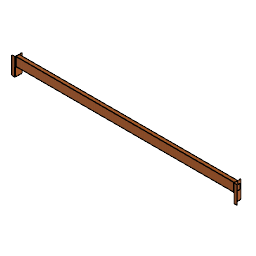
_Cross Bar.9fb02594-36a0-4474-9139-e6fe5210b81d (Autodesk Fusion 360 design; units mm, degrees)
Autodesk Fusion 360 part; units mm, degrees
(part 1 of 2)
sketch "Sketch1" plane through (0, 0, 0) normal (0, 1, 0) x (1, 0, 0)
  line L0 (-1250.95, 0) -> (0, 0)
  line L1 (-1257.3, 6.35) -> (-1257.3, 203.2)
  line L2 (-1257.3, 203.2) -> (-1216.025, 203.2)
  line L3 (-1257.3, 6.35) -> (-1250.95, 0)
  line L4 (-1216.025, 0) -> (-1216.025, 101.6)
  line L5 (-1216.025, 101.6) -> (-1216.025, 203.2)
  line L6 (0, 0) -> (0, -58.9173) construction
  line L7 (-1216.025, 101.6) -> (0, 101.6)
  line L8 (0, 0) -> (0, -58.9173) construction
  line L9 (1216.025, 0) -> (1216.025, 101.6)
  line L10 (1216.025, 101.6) -> (1216.025, 203.2)
  line L11 (1250.95, 0) -> (0, 0)
  line L12 (1257.3, 6.35) -> (1257.3, 203.2)
  line L13 (1257.3, 6.35) -> (1250.95, 0)
  line L14 (1257.3, 203.2) -> (1216.025, 203.2)
  line L15 (1216.025, 101.6) -> (0, 101.6)
  dimension "d3" = 41.275
  dimension "d6" = 101.6
  constraint coincident L0.end L6.start
  constraint horizontal L0
  constraint perpendicular L0 L1
  constraint perpendicular L1 L2
  constraint coincident L0 L6.start
  constraint coincident L0 L4.start
  constraint perpendicular L0 L4
  constraint perpendicular L2 L5
  constraint perpendicular L0 L6
  constraint coincident L6 L0.end
  constraint perpendicular L4 L7
  constraint symmetric L0.end L6 L8.start
  constraint symmetric L1.end L6 L12.end
  constraint symmetric L2.end L6 L10.end
  constraint symmetric L1.start L6 L12.start
  constraint symmetric L0.start L6 L11.start
  constraint symmetric L4.start L6 L9.start
  constraint symmetric L4.end L6 L9.end
  constraint symmetric L8.end L6 L6.end
  constraint symmetric L6 L0.end L8.start
  constraint symmetric L6 L7.end L15.end
  measures "d3" distance of L1.end L2.end
  measures "d6" distance of L4.start L4.end
extrude "Extrude1" add sketch "Sketch1" against normal blind 3.175 contours L0 L1 L2 L3 L4 L5 | L9 L10 L11 L12 L13 L14 makes body 1 at (-1229.7833, 0, -69.85) makes body 2 at (1229.7833, 0, -69.85)
ref_plane "WorkPlane1" through (1236.6625, 3.175, -101.6) normal (0, -1, 0) x (0, 0, -1)
sketch "Sketch2" plane through (0, 3.175, 0) normal (0, -1, 0) x (-1, 0, 0)
  line L0 (-1257.3, 6.35) -> (-1257.3, 203.2)
  line L1 (-1216.025, 0) -> (-1216.025, 101.6)
  line L2 (-1216.025, 101.6) -> (0, 101.6)
  line L3 (-1250.95, 0) -> (0, 0)
  line L4 (-1257.3, 6.35) -> (-1250.95, 0)
  line L5 (-1216.025, 101.6) -> (-1216.025, 203.2)
  line L6 (-1257.3, 203.2) -> (-1216.025, 203.2)
  line L7 (1216.025, 101.6) -> (0, 101.6)
  line L8 (1250.95, 0) -> (0, 0)
  line L9 (1257.3, 6.35) -> (1250.95, 0)
  line L10 (1257.3, 6.35) -> (1257.3, 203.2)
  line L11 (1216.025, 0) -> (1216.025, 101.6)
  line L12 (1257.3, 203.2) -> (1216.025, 203.2)
  line L13 (1216.025, 101.6) -> (1216.025, 203.2)
extrude "Extrude2" add sketch "Sketch2" against normal blind 42.545 separate body contours L1 L2 L3 L7 L8 L11 makes body 3
sketch "Sketch3" plane through (0, 0, 0) normal (0, 0, 1) x (-1, 0, 0)
  line L0 (1216.025, -3.175) -> (-1216.025, -3.175)
  line L1 (-1216.025, -3.175) -> (-1216.025, -45.72)
  line L2 (-1216.025, -45.72) -> (1216.025, -45.72)
  line L3 (1216.025, -45.72) -> (1216.025, -3.175)
  line L4 (-1250.95, 0) -> (-1216.025, 0)
  line L5 (-1216.025, 0) -> (-1216.025, 3.175)
  line L6 (-1216.025, 3.175) -> (-1250.95, 3.175)
  line L7 (-1250.95, 3.175) -> (-1250.95, 0)
  line L8 (-1216.025, -3.175) -> (-1212.215, -3.175)
  line L9 (-1216.025, 3.175) -> (-1212.215, -3.175)
  line L10 (-1216.025, 0) -> (-1216.025, -3.175)
  line L11 (-1250.95, 0) -> (-1250.95, 3.175)
  line L12 (1219.2, -45.72) -> (-1219.2, -45.72)
  line L13 (-1219.2, -45.72) -> (-1219.2, 0)
  line L14 (0, -3.175) -> (0, -45.72)
  line L15 (0, -24.4475) -> (-1216.025, -24.4475)
  line L16 (-1257.3, 3.175) -> (-1250.95, 3.175)
  line L17 (-1257.3, 0) -> (-1257.3, 3.175)
  line L18 (-1257.3, 0) -> (-1250.95, 0)
  line L19 (-1250.95, 0) -> (-1250.95, 3.175)
  line L20 (-1250.95, 3.175) -> (-1257.3, 3.175)
  line L21 (-1257.3, 3.175) -> (-1257.3, 0)
  line L22 (-1216.025, -3.175) -> (1216.025, -3.175)
  line L23 (0, -24.4475) -> (1216.025, -24.4475)
  line L24 (1216.025, -3.175) -> (1216.025, -45.72)
  line L25 (1216.025, 0) -> (1216.025, 3.175)
  line L26 (-1219.2, -45.72) -> (1219.2, -45.72)
  line L27 (1257.3, 0) -> (1250.95, 0)
  line L28 (1216.025, -45.72) -> (-1216.025, -45.72)
  line L29 (1250.95, 3.175) -> (1250.95, 0)
  line L30 (1257.3, 3.175) -> (1250.95, 3.175)
  line L31 (1216.025, -3.175) -> (1212.215, -3.175)
  line L32 (1250.95, 3.175) -> (1257.3, 3.175)
  line L33 (1250.95, 0) -> (1216.025, 0)
  line L34 (1216.025, 3.175) -> (1250.95, 3.175)
  line L35 (1216.025, 3.175) -> (1212.215, -3.175)
  line L36 (1250.95, 0) -> (1250.95, 3.175)
  line L37 (1250.95, 0) -> (1250.95, 3.175)
  line L38 (1216.025, 0) -> (1216.025, -3.175)
  line L39 (1257.3, 0) -> (1257.3, 3.175)
  line L40 (1219.2, -45.72) -> (1219.2, 0)
  line L41 (1257.3, 3.175) -> (1257.3, 0)
  point P0 (0, -45.72)
  dimension "d12" = 3.81
  dimension "d13" = 2438.4
  constraint coincident L0.end L1.start
  constraint perpendicular L1 L8
  constraint coincident L5.end L6.start
  constraint coincident L4.end L5.start
  constraint coincident L4.start L7.end
  constraint coincident L6.end L7.start
  constraint midpoint L12 P0
  constraint coincident L2 P0
  constraint parallel L2 L12
  constraint coincident L4 L13.end
  constraint perpendicular L4 L13
  constraint midpoint L0 L14.start
  constraint coincident P0 L14.end
  constraint perpendicular L12 L14
  constraint midpoint L14 L15.start
  constraint midpoint L1 L15.end
  constraint symmetric L0.start L14 L0.end
  constraint symmetric L0.end L14 L0.start
  constraint symmetric L1.end L14 L2.end
  constraint symmetric L2.end L14 L1.end
  constraint symmetric L4.start L14 L27.end
  constraint symmetric L4.end L14 L25.start
  constraint symmetric L5.end L14 L25.end
  constraint symmetric L6.end L14 L29.start
  constraint symmetric L8.end L14 L31.end
  constraint symmetric L12.start L14 L12.end
  constraint symmetric L12.end L14 L12.start
  constraint symmetric L13.end L14 L40.end
  constraint symmetric L14 L15.start L23.start
  constraint symmetric L14 L15.end L23.end
  constraint symmetric L14 L16.start L30.start
  constraint symmetric L14 L6.end L29.start
  constraint symmetric L14 L17.start L27.start
  constraint symmetric L14 L4.start L27.end
  measures "d12" distance of L0.end L8.end
  measures "d13" distance of L12.start L12.end
extrude "Extrude3" add sketch "Sketch3" against normal blind 203.2 contours L3 L12 L24 L26 L33 L38 L40 | L0 L22 L25 L31 L35 L38 | L0 L5 L8 L9 L10 L22 | L1 L4 L10 L12 L13 L26 bodies 1 2 3
delete_face "DeleteFace1" 1 faces at (1213.485, 3.175, -169.3333) on bodies 1
delete_face "DeleteFace2" 1 faces at (-1214.755, 3.175, -135.4667) on bodies 1
sketch "Sketch4" plane through (0, 45.72, 0) normal (0, 1, 0) x (-1, 0, 0)
  line L0 (1219.2, 0) -> (-1219.2, 0)
  line L1 (-1219.2, 0) -> (-1219.2, -203.2)
  line L2 (-1219.2, -203.2) -> (-1216.025, -203.2)
  line L3 (-1216.025, -203.2) -> (-1216.025, -101.6)
  line L4 (-1216.025, -101.6) -> (1216.025, -101.6)
  line L5 (1216.025, -101.6) -> (1216.025, -203.2)
  line L6 (1216.025, -203.2) -> (1219.2, -203.2)
  line L7 (1219.2, -203.2) -> (1219.2, 0)
  line L8 (0, 0) -> (0, -41.91)
  line L9 (-1219.2, -41.91) -> (1219.2, -41.91)
  line L10 (1216.025, -101.6) -> (1219.2, -101.6)
  line L11 (1219.2, -101.6) -> (-1219.2, -101.6)
  dimension "d16" = 41.91
  constraint coincident L8.start origin
  constraint perpendicular L0 L8
  constraint midpoint L8.end L9
  constraint coincident L7 L9.end
  constraint perpendicular L7 L9
  constraint coincident L4.end L5.start
  constraint midpoint L7 L10.end
  constraint midpoint L1 L11.end
  measures "d16" distance of L8.start L8.end
extrude "Extrude4" add sketch "Sketch4" along normal blind 25.4 contours L1 L4 L7 L9 L10 L11 bodies 1
sketch "Sketch5" plane through (1219.2, 0, 0) normal (1, 0, 0) x (0, 1, 0)
  line L0 (45.72, 0) -> (0, 0)
  line L1 (0, 0) -> (0, -203.2)
  line L2 (0, -203.2) -> (45.72, -203.2)
  line L3 (45.72, -203.2) -> (45.72, -101.6)
  line L4 (45.72, -101.6) -> (71.12, -101.6)
  line L5 (71.12, -101.6) -> (71.12, -41.91)
  line L6 (71.12, -41.91) -> (45.72, -41.91)
  line L7 (45.72, -41.91) -> (45.72, 0)
  line L8 (0, -203.2) -> (0, -6.35)
  line L9 (0, -6.35) -> (-3.175, -6.35)
  line L10 (-3.175, -6.35) -> (-3.175, -203.2)
  line L11 (-3.175, -203.2) -> (0, -203.2)
  line L12 (0, -6.35) -> (0, 0)
  line L13 (0, 0) -> (-3.175, 0)
  line L14 (-3.175, 0) -> (-3.175, -6.35)
  line L15 (-3.175, -6.35) -> (0, -6.35)
  line L16 (-3.175, 0) -> (80.01, 0)
  line L17 (80.01, 0) -> (45.72, 0)
  line L18 (45.72, 0) -> (45.72, -203.2)
  line L19 (45.72, -203.2) -> (80.01, -203.2)
  line L20 (80.01, -203.2) -> (80.01, 0)
  line L21 (80.01, -203.2) -> (80.01, -196.85)
  line L22 (80.01, -203.2) -> (73.66, -203.2)
  line L23 (73.66, -203.2) -> (80.01, -196.85)
  dimension "d19" = 83.185
  dimension "d22" = 6.35
  dimension "d23" = 6.35
  constraint coincident L13.end L14.start
  constraint perpendicular L14 L16
  constraint horizontal L17
  constraint vertical L18
  constraint horizontal L19
  constraint vertical L20
  constraint coincident L2.end L3.start
  constraint perpendicular L19 L21
  constraint perpendicular L20 L22
  measures "d19" distance of L13.end L16.end
  measures "d22" distance of L19.end L21.end
  measures "d23" distance of L19.end L22.end
extrude "Extrude5" add sketch "Sketch5" against normal blind 3.175 contours L3 L4 L5 L6 L7 L16 L17 L18 L19 L20 L23 | L4 L5 L6 L18 bodies 1
sketch "Sketch6" plane through (0, -3.175, 0) normal (0, -1, 0) x (1, 0, 0)
  line L0 (1257.3, -203.2) -> (1257.3, -6.35)
  line L1 (1257.3, -6.35) -> (1250.95, 0)
  line L2 (1250.95, 0) -> (1216.025, 0)
  line L3 (1216.025, 0) -> (1216.025, -101.6)
  line L4 (1216.025, -101.6) -> (1216.025, -203.2)
  line L5 (1216.025, -203.2) -> (1257.3, -203.2)
  line L6 (1257.3, -203.2) -> (1257.3, -196.85)
  line L7 (1257.3, -203.2) -> (1250.95, -203.2)
  line L8 (1250.95, -203.2) -> (1257.3, -196.85)
  dimension "d24" = 6.35
  dimension "d25" = 6.35
  constraint coincident L0.start L5.end
  constraint perpendicular L5 L6
  constraint perpendicular L0 L7
  measures "d24" distance of L0.start L6.end
  measures "d25" distance of L0.start L7.end
extrude "Extrude6" cut sketch "Sketch6" against normal blind 3.175 contours L0 L5 L6 L7 L8 bodies 1
fillet "Fillet1" radius 6.35 2 edges at (1216.025, -3.175, -152.4) (1216.025, -3.175, -50.8) on bodies 1
fillet "Fillet2" radius 3.175 2 edges at (1217.8849, -1.3151, -101.6) (1216.025, 37.1475, -101.6) on bodies 1
fillet "Fillet3" radius 6.35 1 edges at (1212.215, 3.175, -50.8) on bodies 1
sketch "Sketch7" plane through (0, 0, -41.91) normal (0, 0, 1) x (-1, 0, 0)
  line L0 (-1216.025, -45.72) -> (-1216.025, -71.12)
  line L1 (-1216.025, -71.12) -> (1219.2, -71.12)
  line L2 (1219.2, -71.12) -> (1219.2, -45.72)
  line L3 (1219.2, -45.72) -> (-1216.025, -45.72)
  line L4 (-1194.435, -58.42) -> (-1194.435, -71.12) construction
  arc A0 (-1214.1752, 0.092) -> (-1219.6203, 3.175) centre (-1219.6203, -3.175) ccw
  line L5 (-1219.6203, 3.175) -> (-1250.95, 3.175)
  line L6 (-1250.95, 3.175) -> (-1250.95, 0)
  line L7 (-1250.95, 0) -> (-1219.2, 0)
  line L8 (-1219.2, 0) -> (-1219.2, -80.01)
  line L9 (-1219.2, -80.01) -> (-1216.025, -80.01)
  line L10 (-1216.025, -80.01) -> (-1216.025, -45.72)
  line L11 (-1216.025, -45.72) -> (1219.2, -45.72)
  line L12 (1219.2, -45.72) -> (1219.2, 0)
  line L13 (1219.2, 0) -> (1250.95, 0)
  line L14 (1250.95, 0) -> (1250.95, 3.175)
  line L15 (1250.95, 3.175) -> (1216.025, 3.175)
  line L16 (1216.025, 3.175) -> (1212.215, -3.175)
  line L17 (1212.215, -3.175) -> (-1208.6197, -3.175)
  arc A1 (-1214.0648, -0.092) -> (-1208.6197, -3.175) centre (-1208.6197, 3.175) ccw
  line L18 (-1214.0648, -0.092) -> (-1214.1752, 0.092)
  line L19 (-1196.975, -63.5) -> (-1196.975, -50.8)
  line L20 (-1191.895, -63.5) -> (-1191.895, -50.8)
  arc A2 (-1191.895, -50.8) -> (-1196.975, -50.8) centre (-1194.435, -50.8) ccw
  line L21 (-1194.435, -58.42) -> (-1194.435, -57.15) construction
  line L22 (-1194.435, -48.26) -> (-1194.435, -45.72) construction
  arc A3 (-1196.975, -63.5) -> (-1191.895, -63.5) centre (-1194.435, -63.5) ccw
  line L23 (1219.2, -58.42) -> (1200.15, -58.42)
  line L24 (-1168.9877, -58.42) -> (-1168.9877, -57.15) construction
  line L25 (-1166.4477, -63.5) -> (-1166.4477, -50.8)
  line L26 (-1171.5277, -63.5) -> (-1171.5277, -50.8)
  arc A4 (-1171.5277, -63.5) -> (-1166.4477, -63.5) centre (-1168.9877, -63.5) ccw
  arc A5 (-1166.4477, -50.8) -> (-1171.5277, -50.8) centre (-1168.9877, -50.8) ccw
  line L27 (-1143.5404, -58.42) -> (-1143.5404, -57.15) construction
  line L28 (-1141.0004, -63.5) -> (-1141.0004, -50.8)
  line L29 (-1146.0804, -63.5) -> (-1146.0804, -50.8)
  arc A6 (-1146.0804, -63.5) -> (-1141.0004, -63.5) centre (-1143.5404, -63.5) ccw
  arc A7 (-1141.0004, -50.8) -> (-1146.0804, -50.8) centre (-1143.5404, -50.8) ccw
  line L30 (-1118.0931, -58.42) -> (-1118.0931, -57.15) construction
  line L31 (-1115.5531, -63.5) -> (-1115.5531, -50.8)
  line L32 (-1120.6331, -63.5) -> (-1120.6331, -50.8)
  arc A8 (-1120.6331, -63.5) -> (-1115.5531, -63.5) centre (-1118.0931, -63.5) ccw
  arc A9 (-1115.5531, -50.8) -> (-1120.6331, -50.8) centre (-1118.0931, -50.8) ccw
  line L33 (-1092.6459, -58.42) -> (-1092.6459, -57.15) construction
  line L34 (-1090.1059, -63.5) -> (-1090.1059, -50.8)
  line L35 (-1095.1859, -63.5) -> (-1095.1859, -50.8)
  arc A10 (-1095.1859, -63.5) -> (-1090.1059, -63.5) centre (-1092.6459, -63.5) ccw
  arc A11 (-1090.1059, -50.8) -> (-1095.1859, -50.8) centre (-1092.6459, -50.8) ccw
  line L36 (-1067.1986, -58.42) -> (-1067.1986, -57.15) construction
  line L37 (-1064.6586, -63.5) -> (-1064.6586, -50.8)
  line L38 (-1069.7386, -63.5) -> (-1069.7386, -50.8)
  arc A12 (-1069.7386, -63.5) -> (-1064.6586, -63.5) centre (-1067.1986, -63.5) ccw
  arc A13 (-1064.6586, -50.8) -> (-1069.7386, -50.8) centre (-1067.1986, -50.8) ccw
  line L39 (-1041.7513, -58.42) -> (-1041.7513, -57.15) construction
  line L40 (-1039.2113, -63.5) -> (-1039.2113, -50.8)
  line L41 (-1044.2913, -63.5) -> (-1044.2913, -50.8)
  arc A14 (-1044.2913, -63.5) -> (-1039.2113, -63.5) centre (-1041.7513, -63.5) ccw
  arc A15 (-1039.2113, -50.8) -> (-1044.2913, -50.8) centre (-1041.7513, -50.8) ccw
  line L42 (-1016.304, -58.42) -> (-1016.304, -57.15) construction
  line L43 (-1013.764, -63.5) -> (-1013.764, -50.8)
  line L44 (-1018.844, -63.5) -> (-1018.844, -50.8)
  arc A16 (-1018.844, -63.5) -> (-1013.764, -63.5) centre (-1016.304, -63.5) ccw
  arc A17 (-1013.764, -50.8) -> (-1018.844, -50.8) centre (-1016.304, -50.8) ccw
  line L45 (-990.8567, -58.42) -> (-990.8567, -57.15) construction
  line L46 (-988.3167, -63.5) -> (-988.3167, -50.8)
  line L47 (-993.3967, -63.5) -> (-993.3967, -50.8)
  arc A18 (-993.3967, -63.5) -> (-988.3167, -63.5) centre (-990.8567, -63.5) ccw
  arc A19 (-988.3167, -50.8) -> (-993.3967, -50.8) centre (-990.8567, -50.8) ccw
  line L48 (-965.4094, -58.42) -> (-965.4094, -57.15) construction
  line L49 (-962.8694, -63.5) -> (-962.8694, -50.8)
  line L50 (-967.9494, -63.5) -> (-967.9494, -50.8)
  arc A20 (-967.9494, -63.5) -> (-962.8694, -63.5) centre (-965.4094, -63.5) ccw
  arc A21 (-962.8694, -50.8) -> (-967.9494, -50.8) centre (-965.4094, -50.8) ccw
  line L51 (-939.9621, -58.42) -> (-939.9621, -57.15) construction
  line L52 (-937.4221, -63.5) -> (-937.4221, -50.8)
  line L53 (-942.5021, -63.5) -> (-942.5021, -50.8)
  arc A22 (-942.5021, -63.5) -> (-937.4221, -63.5) centre (-939.9621, -63.5) ccw
  arc A23 (-937.4221, -50.8) -> (-942.5021, -50.8) centre (-939.9621, -50.8) ccw
  line L54 (-914.5148, -58.42) -> (-914.5148, -57.15) construction
  line L55 (-911.9748, -63.5) -> (-911.9748, -50.8)
  line L56 (-917.0548, -63.5) -> (-917.0548, -50.8)
  arc A24 (-917.0548, -63.5) -> (-911.9748, -63.5) centre (-914.5148, -63.5) ccw
  arc A25 (-911.9748, -50.8) -> (-917.0548, -50.8) centre (-914.5148, -50.8) ccw
  line L57 (-889.0676, -58.42) -> (-889.0676, -57.15) construction
  line L58 (-886.5276, -63.5) -> (-886.5276, -50.8)
  line L59 (-891.6076, -63.5) -> (-891.6076, -50.8)
  arc A26 (-891.6076, -63.5) -> (-886.5276, -63.5) centre (-889.0676, -63.5) ccw
  arc A27 (-886.5276, -50.8) -> (-891.6076, -50.8) centre (-889.0676, -50.8) ccw
  line L60 (-863.6203, -58.42) -> (-863.6203, -57.15) construction
  line L61 (-861.0803, -63.5) -> (-861.0803, -50.8)
  line L62 (-866.1603, -63.5) -> (-866.1603, -50.8)
  arc A28 (-866.1603, -63.5) -> (-861.0803, -63.5) centre (-863.6203, -63.5) ccw
  arc A29 (-861.0803, -50.8) -> (-866.1603, -50.8) centre (-863.6203, -50.8) ccw
  line L63 (-838.173, -58.42) -> (-838.173, -57.15) construction
  line L64 (-835.633, -63.5) -> (-835.633, -50.8)
  line L65 (-840.713, -63.5) -> (-840.713, -50.8)
  arc A30 (-840.713, -63.5) -> (-835.633, -63.5) centre (-838.173, -63.5) ccw
  arc A31 (-835.633, -50.8) -> (-840.713, -50.8) centre (-838.173, -50.8) ccw
  line L66 (-812.7257, -58.42) -> (-812.7257, -57.15) construction
  line L67 (-810.1857, -63.5) -> (-810.1857, -50.8)
  line L68 (-815.2657, -63.5) -> (-815.2657, -50.8)
  arc A32 (-815.2657, -63.5) -> (-810.1857, -63.5) centre (-812.7257, -63.5) ccw
  arc A33 (-810.1857, -50.8) -> (-815.2657, -50.8) centre (-812.7257, -50.8) ccw
  line L69 (-787.2784, -58.42) -> (-787.2784, -57.15) construction
  line L70 (-784.7384, -63.5) -> (-784.7384, -50.8)
  line L71 (-789.8184, -63.5) -> (-789.8184, -50.8)
  arc A34 (-789.8184, -63.5) -> (-784.7384, -63.5) centre (-787.2784, -63.5) ccw
  arc A35 (-784.7384, -50.8) -> (-789.8184, -50.8) centre (-787.2784, -50.8) ccw
  line L72 (-761.8311, -58.42) -> (-761.8311, -57.15) construction
  line L73 (-759.2911, -63.5) -> (-759.2911, -50.8)
  line L74 (-764.3711, -63.5) -> (-764.3711, -50.8)
  arc A36 (-764.3711, -63.5) -> (-759.2911, -63.5) centre (-761.8311, -63.5) ccw
  arc A37 (-759.2911, -50.8) -> (-764.3711, -50.8) centre (-761.8311, -50.8) ccw
  line L75 (-736.3838, -58.42) -> (-736.3838, -57.15) construction
  line L76 (-733.8438, -63.5) -> (-733.8438, -50.8)
  line L77 (-738.9238, -63.5) -> (-738.9238, -50.8)
  arc A38 (-738.9238, -63.5) -> (-733.8438, -63.5) centre (-736.3838, -63.5) ccw
  arc A39 (-733.8438, -50.8) -> (-738.9238, -50.8) centre (-736.3838, -50.8) ccw
  line L78 (-710.9365, -58.42) -> (-710.9365, -57.15) construction
  line L79 (-708.3965, -63.5) -> (-708.3965, -50.8)
  line L80 (-713.4765, -63.5) -> (-713.4765, -50.8)
  arc A40 (-713.4765, -63.5) -> (-708.3965, -63.5) centre (-710.9365, -63.5) ccw
  arc A41 (-708.3965, -50.8) -> (-713.4765, -50.8) centre (-710.9365, -50.8) ccw
  line L81 (-685.4893, -58.42) -> (-685.4893, -57.15) construction
  line L82 (-682.9493, -63.5) -> (-682.9493, -50.8)
  line L83 (-688.0293, -63.5) -> (-688.0293, -50.8)
  arc A42 (-688.0293, -63.5) -> (-682.9493, -63.5) centre (-685.4893, -63.5) ccw
  arc A43 (-682.9493, -50.8) -> (-688.0293, -50.8) centre (-685.4893, -50.8) ccw
  line L84 (-660.042, -58.42) -> (-660.042, -57.15) construction
  line L85 (-657.502, -63.5) -> (-657.502, -50.8)
  line L86 (-662.582, -63.5) -> (-662.582, -50.8)
  arc A44 (-662.582, -63.5) -> (-657.502, -63.5) centre (-660.042, -63.5) ccw
  arc A45 (-657.502, -50.8) -> (-662.582, -50.8) centre (-660.042, -50.8) ccw
  line L87 (-634.5947, -58.42) -> (-634.5947, -57.15) construction
  line L88 (-632.0547, -63.5) -> (-632.0547, -50.8)
  line L89 (-637.1347, -63.5) -> (-637.1347, -50.8)
  arc A46 (-637.1347, -63.5) -> (-632.0547, -63.5) centre (-634.5947, -63.5) ccw
  arc A47 (-632.0547, -50.8) -> (-637.1347, -50.8) centre (-634.5947, -50.8) ccw
  line L90 (-609.1474, -58.42) -> (-609.1474, -57.15) construction
  line L91 (-606.6074, -63.5) -> (-606.6074, -50.8)
  line L92 (-611.6874, -63.5) -> (-611.6874, -50.8)
  arc A48 (-611.6874, -63.5) -> (-606.6074, -63.5) centre (-609.1474, -63.5) ccw
  arc A49 (-606.6074, -50.8) -> (-611.6874, -50.8) centre (-609.1474, -50.8) ccw
  line L93 (-583.7001, -58.42) -> (-583.7001, -57.15) construction
  line L94 (-581.1601, -63.5) -> (-581.1601, -50.8)
  line L95 (-586.2401, -63.5) -> (-586.2401, -50.8)
  arc A50 (-586.2401, -63.5) -> (-581.1601, -63.5) centre (-583.7001, -63.5) ccw
  arc A51 (-581.1601, -50.8) -> (-586.2401, -50.8) centre (-583.7001, -50.8) ccw
  line L96 (-558.2528, -58.42) -> (-558.2528, -57.15) construction
  line L97 (-555.7128, -63.5) -> (-555.7128, -50.8)
  line L98 (-560.7928, -63.5) -> (-560.7928, -50.8)
  arc A52 (-560.7928, -63.5) -> (-555.7128, -63.5) centre (-558.2528, -63.5) ccw
  arc A53 (-555.7128, -50.8) -> (-560.7928, -50.8) centre (-558.2528, -50.8) ccw
  line L99 (-532.8055, -58.42) -> (-532.8055, -57.15) construction
  line L100 (-530.2655, -63.5) -> (-530.2655, -50.8)
  line L101 (-535.3455, -63.5) -> (-535.3455, -50.8)
  arc A54 (-535.3455, -63.5) -> (-530.2655, -63.5) centre (-532.8055, -63.5) ccw
  arc A55 (-530.2655, -50.8) -> (-535.3455, -50.8) centre (-532.8055, -50.8) ccw
  line L102 (-507.3582, -58.42) -> (-507.3582, -57.15) construction
  line L103 (-504.8182, -63.5) -> (-504.8182, -50.8)
  line L104 (-509.8982, -63.5) -> (-509.8982, -50.8)
  arc A56 (-509.8982, -63.5) -> (-504.8182, -63.5) centre (-507.3582, -63.5) ccw
  arc A57 (-504.8182, -50.8) -> (-509.8982, -50.8) centre (-507.3582, -50.8) ccw
  line L105 (-481.911, -58.42) -> (-481.911, -57.15) construction
  line L106 (-479.371, -63.5) -> (-479.371, -50.8)
  line L107 (-484.451, -63.5) -> (-484.451, -50.8)
  arc A58 (-484.451, -63.5) -> (-479.371, -63.5) centre (-481.911, -63.5) ccw
  arc A59 (-479.371, -50.8) -> (-484.451, -50.8) centre (-481.911, -50.8) ccw
  line L108 (-456.4637, -58.42) -> (-456.4637, -57.15) construction
  line L109 (-453.9237, -63.5) -> (-453.9237, -50.8)
  line L110 (-459.0037, -63.5) -> (-459.0037, -50.8)
  arc A60 (-459.0037, -63.5) -> (-453.9237, -63.5) centre (-456.4637, -63.5) ccw
  arc A61 (-453.9237, -50.8) -> (-459.0037, -50.8) centre (-456.4637, -50.8) ccw
  line L111 (-431.0164, -58.42) -> (-431.0164, -57.15) construction
  line L112 (-428.4764, -63.5) -> (-428.4764, -50.8)
  line L113 (-433.5564, -63.5) -> (-433.5564, -50.8)
  arc A62 (-433.5564, -63.5) -> (-428.4764, -63.5) centre (-431.0164, -63.5) ccw
  arc A63 (-428.4764, -50.8) -> (-433.5564, -50.8) centre (-431.0164, -50.8) ccw
  line L114 (-405.5691, -58.42) -> (-405.5691, -57.15) construction
  line L115 (-403.0291, -63.5) -> (-403.0291, -50.8)
  line L116 (-408.1091, -63.5) -> (-408.1091, -50.8)
  arc A64 (-408.1091, -63.5) -> (-403.0291, -63.5) centre (-405.5691, -63.5) ccw
  arc A65 (-403.0291, -50.8) -> (-408.1091, -50.8) centre (-405.5691, -50.8) ccw
  line L117 (-380.1218, -58.42) -> (-380.1218, -57.15) construction
  line L118 (-377.5818, -63.5) -> (-377.5818, -50.8)
  line L119 (-382.6618, -63.5) -> (-382.6618, -50.8)
  arc A66 (-382.6618, -63.5) -> (-377.5818, -63.5) centre (-380.1218, -63.5) ccw
  arc A67 (-377.5818, -50.8) -> (-382.6618, -50.8) centre (-380.1218, -50.8) ccw
  line L120 (-354.6745, -58.42) -> (-354.6745, -57.15) construction
  line L121 (-352.1345, -63.5) -> (-352.1345, -50.8)
  line L122 (-357.2145, -63.5) -> (-357.2145, -50.8)
  arc A68 (-357.2145, -63.5) -> (-352.1345, -63.5) centre (-354.6745, -63.5) ccw
  arc A69 (-352.1345, -50.8) -> (-357.2145, -50.8) centre (-354.6745, -50.8) ccw
  line L123 (-329.2272, -58.42) -> (-329.2272, -57.15) construction
  line L124 (-326.6872, -63.5) -> (-326.6872, -50.8)
  line L125 (-331.7672, -63.5) -> (-331.7672, -50.8)
  arc A70 (-331.7672, -63.5) -> (-326.6872, -63.5) centre (-329.2272, -63.5) ccw
  arc A71 (-326.6872, -50.8) -> (-331.7672, -50.8) centre (-329.2272, -50.8) ccw
  line L126 (-303.7799, -58.42) -> (-303.7799, -57.15) construction
  line L127 (-301.2399, -63.5) -> (-301.2399, -50.8)
  line L128 (-306.3199, -63.5) -> (-306.3199, -50.8)
  arc A72 (-306.3199, -63.5) -> (-301.2399, -63.5) centre (-303.7799, -63.5) ccw
  arc A73 (-301.2399, -50.8) -> (-306.3199, -50.8) centre (-303.7799, -50.8) ccw
  line L129 (-278.3327, -58.42) -> (-278.3327, -57.15) construction
  line L130 (-275.7927, -63.5) -> (-275.7927, -50.8)
  line L131 (-280.8727, -63.5) -> (-280.8727, -50.8)
  arc A74 (-280.8727, -63.5) -> (-275.7927, -63.5) centre (-278.3327, -63.5) ccw
  arc A75 (-275.7927, -50.8) -> (-280.8727, -50.8) centre (-278.3327, -50.8) ccw
  line L132 (-252.8854, -58.42) -> (-252.8854, -57.15) construction
  line L133 (-250.3454, -63.5) -> (-250.3454, -50.8)
  line L134 (-255.4254, -63.5) -> (-255.4254, -50.8)
  arc A76 (-255.4254, -63.5) -> (-250.3454, -63.5) centre (-252.8854, -63.5) ccw
  arc A77 (-250.3454, -50.8) -> (-255.4254, -50.8) centre (-252.8854, -50.8) ccw
  line L135 (-227.4381, -58.42) -> (-227.4381, -57.15) construction
  line L136 (-224.8981, -63.5) -> (-224.8981, -50.8)
  line L137 (-229.9781, -63.5) -> (-229.9781, -50.8)
  arc A78 (-229.9781, -63.5) -> (-224.8981, -63.5) centre (-227.4381, -63.5) ccw
  arc A79 (-224.8981, -50.8) -> (-229.9781, -50.8) centre (-227.4381, -50.8) ccw
  line L138 (-201.9908, -58.42) -> (-201.9908, -57.15) construction
  line L139 (-199.4508, -63.5) -> (-199.4508, -50.8)
  line L140 (-204.5308, -63.5) -> (-204.5308, -50.8)
  arc A80 (-204.5308, -63.5) -> (-199.4508, -63.5) centre (-201.9908, -63.5) ccw
  arc A81 (-199.4508, -50.8) -> (-204.5308, -50.8) centre (-201.9908, -50.8) ccw
  line L141 (-176.5435, -58.42) -> (-176.5435, -57.15) construction
  line L142 (-174.0035, -63.5) -> (-174.0035, -50.8)
  line L143 (-179.0835, -63.5) -> (-179.0835, -50.8)
  arc A82 (-179.0835, -63.5) -> (-174.0035, -63.5) centre (-176.5435, -63.5) ccw
  arc A83 (-174.0035, -50.8) -> (-179.0835, -50.8) centre (-176.5435, -50.8) ccw
  line L144 (-151.0962, -58.42) -> (-151.0962, -57.15) construction
  line L145 (-148.5562, -63.5) -> (-148.5562, -50.8)
  line L146 (-153.6362, -63.5) -> (-153.6362, -50.8)
  arc A84 (-153.6362, -63.5) -> (-148.5562, -63.5) centre (-151.0962, -63.5) ccw
  arc A85 (-148.5562, -50.8) -> (-153.6362, -50.8) centre (-151.0962, -50.8) ccw
  line L147 (-125.6489, -58.42) -> (-125.6489, -57.15) construction
  line L148 (-123.1089, -63.5) -> (-123.1089, -50.8)
  line L149 (-128.1889, -63.5) -> (-128.1889, -50.8)
  arc A86 (-128.1889, -63.5) -> (-123.1089, -63.5) centre (-125.6489, -63.5) ccw
  arc A87 (-123.1089, -50.8) -> (-128.1889, -50.8) centre (-125.6489, -50.8) ccw
  line L150 (-100.2016, -58.42) -> (-100.2016, -57.15) construction
  line L151 (-97.6616, -63.5) -> (-97.6616, -50.8)
  line L152 (-102.7416, -63.5) -> (-102.7416, -50.8)
  arc A88 (-102.7416, -63.5) -> (-97.6616, -63.5) centre (-100.2016, -63.5) ccw
  arc A89 (-97.6616, -50.8) -> (-102.7416, -50.8) centre (-100.2016, -50.8) ccw
  line L153 (-74.7544, -58.42) -> (-74.7544, -57.15) construction
  line L154 (-72.2144, -63.5) -> (-72.2144, -50.8)
  line L155 (-77.2944, -63.5) -> (-77.2944, -50.8)
  arc A90 (-77.2944, -63.5) -> (-72.2144, -63.5) centre (-74.7544, -63.5) ccw
  arc A91 (-72.2144, -50.8) -> (-77.2944, -50.8) centre (-74.7544, -50.8) ccw
  line L156 (-49.3071, -58.42) -> (-49.3071, -57.15) construction
  line L157 (-46.7671, -63.5) -> (-46.7671, -50.8)
  line L158 (-51.8471, -63.5) -> (-51.8471, -50.8)
  arc A92 (-51.8471, -63.5) -> (-46.7671, -63.5) centre (-49.3071, -63.5) ccw
  arc A93 (-46.7671, -50.8) -> (-51.8471, -50.8) centre (-49.3071, -50.8) ccw
  line L159 (-23.8598, -58.42) -> (-23.8598, -57.15) construction
  line L160 (-21.3198, -63.5) -> (-21.3198, -50.8)
  line L161 (-26.3998, -63.5) -> (-26.3998, -50.8)
  arc A94 (-26.3998, -63.5) -> (-21.3198, -63.5) centre (-23.8598, -63.5) ccw
  arc A95 (-21.3198, -50.8) -> (-26.3998, -50.8) centre (-23.8598, -50.8) ccw
  line L162 (1.5875, -58.42) -> (1.5875, -57.15) construction
  line L163 (4.1275, -63.5) -> (4.1275, -50.8)
  line L164 (-0.9525, -63.5) -> (-0.9525, -50.8)
  arc A96 (-0.9525, -63.5) -> (4.1275, -63.5) centre (1.5875, -63.5) ccw
  arc A97 (4.1275, -50.8) -> (-0.9525, -50.8) centre (1.5875, -50.8) ccw
  line L165 (27.0348, -58.42) -> (27.0348, -57.15) construction
  line L166 (29.5748, -63.5) -> (29.5748, -50.8)
  line L167 (24.4948, -63.5) -> (24.4948, -50.8)
  arc A98 (24.4948, -63.5) -> (29.5748, -63.5) centre (27.0348, -63.5) ccw
  arc A99 (29.5748, -50.8) -> (24.4948, -50.8) centre (27.0348, -50.8) ccw
  line L168 (52.4821, -58.42) -> (52.4821, -57.15) construction
  line L169 (55.0221, -63.5) -> (55.0221, -50.8)
  line L170 (49.9421, -63.5) -> (49.9421, -50.8)
  arc A100 (49.9421, -63.5) -> (55.0221, -63.5) centre (52.4821, -63.5) ccw
  arc A101 (55.0221, -50.8) -> (49.9421, -50.8) centre (52.4821, -50.8) ccw
  line L171 (77.9294, -58.42) -> (77.9294, -57.15) construction
  line L172 (80.4694, -63.5) -> (80.4694, -50.8)
  line L173 (75.3894, -63.5) -> (75.3894, -50.8)
  arc A102 (75.3894, -63.5) -> (80.4694, -63.5) centre (77.9294, -63.5) ccw
  arc A103 (80.4694, -50.8) -> (75.3894, -50.8) centre (77.9294, -50.8) ccw
  line L174 (103.3766, -58.42) -> (103.3766, -57.15) construction
  line L175 (105.9166, -63.5) -> (105.9166, -50.8)
  line L176 (100.8366, -63.5) -> (100.8366, -50.8)
  arc A104 (100.8366, -63.5) -> (105.9166, -63.5) centre (103.3766, -63.5) ccw
  arc A105 (105.9166, -50.8) -> (100.8366, -50.8) centre (103.3766, -50.8) ccw
  line L177 (128.8239, -58.42) -> (128.8239, -57.15) construction
  line L178 (131.3639, -63.5) -> (131.3639, -50.8)
  line L179 (126.2839, -63.5) -> (126.2839, -50.8)
  arc A106 (126.2839, -63.5) -> (131.3639, -63.5) centre (128.8239, -63.5) ccw
  arc A107 (131.3639, -50.8) -> (126.2839, -50.8) centre (128.8239, -50.8) ccw
  line L180 (154.2712, -58.42) -> (154.2712, -57.15) construction
  line L181 (156.8112, -63.5) -> (156.8112, -50.8)
  line L182 (151.7312, -63.5) -> (151.7312, -50.8)
  arc A108 (151.7312, -63.5) -> (156.8112, -63.5) centre (154.2712, -63.5) ccw
  arc A109 (156.8112, -50.8) -> (151.7312, -50.8) centre (154.2712, -50.8) ccw
  line L183 (179.7185, -58.42) -> (179.7185, -57.15) construction
  line L184 (182.2585, -63.5) -> (182.2585, -50.8)
  line L185 (177.1785, -63.5) -> (177.1785, -50.8)
  arc A110 (177.1785, -63.5) -> (182.2585, -63.5) centre (179.7185, -63.5) ccw
  arc A111 (182.2585, -50.8) -> (177.1785, -50.8) centre (179.7185, -50.8) ccw
  line L186 (205.1658, -58.42) -> (205.1658, -57.15) construction
  line L187 (207.7058, -63.5) -> (207.7058, -50.8)
  line L188 (202.6258, -63.5) -> (202.6258, -50.8)
  arc A112 (202.6258, -63.5) -> (207.7058, -63.5) centre (205.1658, -63.5) ccw
  arc A113 (207.7058, -50.8) -> (202.6258, -50.8) centre (205.1658, -50.8) ccw
  line L189 (230.6131, -58.42) -> (230.6131, -57.15) construction
  line L190 (233.1531, -63.5) -> (233.1531, -50.8)
  line L191 (228.0731, -63.5) -> (228.0731, -50.8)
  arc A114 (228.0731, -63.5) -> (233.1531, -63.5) centre (230.6131, -63.5) ccw
  arc A115 (233.1531, -50.8) -> (228.0731, -50.8) centre (230.6131, -50.8) ccw
  line L192 (256.0604, -58.42) -> (256.0604, -57.15) construction
  line L193 (258.6004, -63.5) -> (258.6004, -50.8)
  line L194 (253.5204, -63.5) -> (253.5204, -50.8)
  arc A116 (253.5204, -63.5) -> (258.6004, -63.5) centre (256.0604, -63.5) ccw
  arc A117 (258.6004, -50.8) -> (253.5204, -50.8) centre (256.0604, -50.8) ccw
  line L195 (281.5077, -58.42) -> (281.5077, -57.15) construction
  line L196 (284.0477, -63.5) -> (284.0477, -50.8)
  line L197 (278.9677, -63.5) -> (278.9677, -50.8)
  arc A118 (278.9677, -63.5) -> (284.0477, -63.5) centre (281.5077, -63.5) ccw
  arc A119 (284.0477, -50.8) -> (278.9677, -50.8) centre (281.5077, -50.8) ccw
  line L198 (306.9549, -58.42) -> (306.9549, -57.15) construction
  line L199 (309.4949, -63.5) -> (309.4949, -50.8)
  line L200 (304.4149, -63.5) -> (304.4149, -50.8)
  arc A120 (304.4149, -63.5) -> (309.4949, -63.5) centre (306.9549, -63.5) ccw
  arc A121 (309.4949, -50.8) -> (304.4149, -50.8) centre (306.9549, -50.8) ccw
  line L201 (332.4022, -58.42) -> (332.4022, -57.15) construction
  line L202 (334.9422, -63.5) -> (334.9422, -50.8)
  line L203 (329.8622, -63.5) -> (329.8622, -50.8)
  arc A122 (329.8622, -63.5) -> (334.9422, -63.5) centre (332.4022, -63.5) ccw
  arc A123 (334.9422, -50.8) -> (329.8622, -50.8) centre (332.4022, -50.8) ccw
  line L204 (357.8495, -58.42) -> (357.8495, -57.15) construction
  line L205 (360.3895, -63.5) -> (360.3895, -50.8)
  line L206 (355.3095, -63.5) -> (355.3095, -50.8)
  arc A124 (355.3095, -63.5) -> (360.3895, -63.5) centre (357.8495, -63.5) ccw
  arc A125 (360.3895, -50.8) -> (355.3095, -50.8) centre (357.8495, -50.8) ccw
  line L207 (383.2968, -58.42) -> (383.2968, -57.15) construction
  line L208 (385.8368, -63.5) -> (385.8368, -50.8)
  line L209 (380.7568, -63.5) -> (380.7568, -50.8)
  arc A126 (380.7568, -63.5) -> (385.8368, -63.5) centre (383.2968, -63.5) ccw
  arc A127 (385.8368, -50.8) -> (380.7568, -50.8) centre (383.2968, -50.8) ccw
  line L210 (408.7441, -58.42) -> (408.7441, -57.15) construction
  line L211 (411.2841, -63.5) -> (411.2841, -50.8)
  line L212 (406.2041, -63.5) -> (406.2041, -50.8)
  arc A128 (406.2041, -63.5) -> (411.2841, -63.5) centre (408.7441, -63.5) ccw
  arc A129 (411.2841, -50.8) -> (406.2041, -50.8) centre (408.7441, -50.8) ccw
  line L213 (434.1914, -58.42) -> (434.1914, -57.15) construction
  line L214 (436.7314, -63.5) -> (436.7314, -50.8)
  line L215 (431.6514, -63.5) -> (431.6514, -50.8)
  arc A130 (431.6514, -63.5) -> (436.7314, -63.5) centre (434.1914, -63.5) ccw
  arc A131 (436.7314, -50.8) -> (431.6514, -50.8) centre (434.1914, -50.8) ccw
  line L216 (459.6387, -58.42) -> (459.6387, -57.15) construction
  line L217 (462.1787, -63.5) -> (462.1787, -50.8)
  line L218 (457.0987, -63.5) -> (457.0987, -50.8)
  arc A132 (457.0987, -63.5) -> (462.1787, -63.5) centre (459.6387, -63.5) ccw
  arc A133 (462.1787, -50.8) -> (457.0987, -50.8) centre (459.6387, -50.8) ccw
  line L219 (485.086, -58.42) -> (485.086, -57.15) construction
  line L220 (487.626, -63.5) -> (487.626, -50.8)
  line L221 (482.546, -63.5) -> (482.546, -50.8)
  arc A134 (482.546, -63.5) -> (487.626, -63.5) centre (485.086, -63.5) ccw
  arc A135 (487.626, -50.8) -> (482.546, -50.8) centre (485.086, -50.8) ccw
  line L222 (510.5332, -58.42) -> (510.5332, -57.15) construction
  line L223 (513.0732, -63.5) -> (513.0732, -50.8)
  line L224 (507.9932, -63.5) -> (507.9932, -50.8)
  arc A136 (507.9932, -63.5) -> (513.0732, -63.5) centre (510.5332, -63.5) ccw
  arc A137 (513.0732, -50.8) -> (507.9932, -50.8) centre (510.5332, -50.8) ccw
  line L225 (535.9805, -58.42) -> (535.9805, -57.15) construction
  line L226 (538.5205, -63.5) -> (538.5205, -50.8)
  line L227 (533.4405, -63.5) -> (533.4405, -50.8)
  arc A138 (533.4405, -63.5) -> (538.5205, -63.5) centre (535.9805, -63.5) ccw
  arc A139 (538.5205, -50.8) -> (533.4405, -50.8) centre (535.9805, -50.8) ccw
  line L228 (561.4278, -58.42) -> (561.4278, -57.15) construction
  line L229 (563.9678, -63.5) -> (563.9678, -50.8)
  line L230 (558.8878, -63.5) -> (558.8878, -50.8)
  arc A140 (558.8878, -63.5) -> (563.9678, -63.5) centre (561.4278, -63.5) ccw
  arc A141 (563.9678, -50.8) -> (558.8878, -50.8) centre (561.4278, -50.8) ccw
  line L231 (586.8751, -58.42) -> (586.8751, -57.15) construction
  line L232 (589.4151, -63.5) -> (589.4151, -50.8)
  line L233 (584.3351, -63.5) -> (584.3351, -50.8)
  arc A142 (584.3351, -63.5) -> (589.4151, -63.5) centre (586.8751, -63.5) ccw
  arc A143 (589.4151, -50.8) -> (584.3351, -50.8) centre (586.8751, -50.8) ccw
  line L234 (612.3224, -58.42) -> (612.3224, -57.15) construction
  line L235 (614.8624, -63.5) -> (614.8624, -50.8)
  line L236 (609.7824, -63.5) -> (609.7824, -50.8)
  arc A144 (609.7824, -63.5) -> (614.8624, -63.5) centre (612.3224, -63.5) ccw
  arc A145 (614.8624, -50.8) -> (609.7824, -50.8) centre (612.3224, -50.8) ccw
  line L237 (637.7697, -58.42) -> (637.7697, -57.15) construction
  line L238 (640.3097, -63.5) -> (640.3097, -50.8)
  line L239 (635.2297, -63.5) -> (635.2297, -50.8)
  arc A146 (635.2297, -63.5) -> (640.3097, -63.5) centre (637.7697, -63.5) ccw
  arc A147 (640.3097, -50.8) -> (635.2297, -50.8) centre (637.7697, -50.8) ccw
  line L240 (663.217, -58.42) -> (663.217, -57.15) construction
  line L241 (665.757, -63.5) -> (665.757, -50.8)
  line L242 (660.677, -63.5) -> (660.677, -50.8)
  arc A148 (660.677, -63.5) -> (665.757, -63.5) centre (663.217, -63.5) ccw
  arc A149 (665.757, -50.8) -> (660.677, -50.8) centre (663.217, -50.8) ccw
  line L243 (688.6643, -58.42) -> (688.6643, -57.15) construction
  line L244 (691.2043, -63.5) -> (691.2043, -50.8)
  line L245 (686.1243, -63.5) -> (686.1243, -50.8)
  arc A150 (686.1243, -63.5) -> (691.2043, -63.5) centre (688.6643, -63.5) ccw
  arc A151 (691.2043, -50.8) -> (686.1243, -50.8) centre (688.6643, -50.8) ccw
  line L246 (714.1115, -58.42) -> (714.1115, -57.15) construction
  line L247 (716.6515, -63.5) -> (716.6515, -50.8)
  line L248 (711.5715, -63.5) -> (711.5715, -50.8)
  arc A152 (711.5715, -63.5) -> (716.6515, -63.5) centre (714.1115, -63.5) ccw
  arc A153 (716.6515, -50.8) -> (711.5715, -50.8) centre (714.1115, -50.8) ccw
  line L249 (739.5588, -58.42) -> (739.5588, -57.15) construction
  line L250 (742.0988, -63.5) -> (742.0988, -50.8)
  line L251 (737.0188, -63.5) -> (737.0188, -50.8)
  arc A154 (737.0188, -63.5) -> (742.0988, -63.5) centre (739.5588, -63.5) ccw
  arc A155 (742.0988, -50.8) -> (737.0188, -50.8) centre (739.5588, -50.8) ccw
  line L252 (765.0061, -58.42) -> (765.0061, -57.15) construction
  line L253 (767.5461, -63.5) -> (767.5461, -50.8)
  line L254 (762.4661, -63.5) -> (762.4661, -50.8)
  arc A156 (762.4661, -63.5) -> (767.5461, -63.5) centre (765.0061, -63.5) ccw
  arc A157 (767.5461, -50.8) -> (762.4661, -50.8) centre (765.0061, -50.8) ccw
  line L255 (790.4534, -58.42) -> (790.4534, -57.15) construction
  line L256 (792.9934, -63.5) -> (792.9934, -50.8)
  line L257 (787.9134, -63.5) -> (787.9134, -50.8)
  arc A158 (787.9134, -63.5) -> (792.9934, -63.5) centre (790.4534, -63.5) ccw
  arc A159 (792.9934, -50.8) -> (787.9134, -50.8) centre (790.4534, -50.8) ccw
  line L258 (815.9007, -58.42) -> (815.9007, -57.15) construction
  line L259 (818.4407, -63.5) -> (818.4407, -50.8)
  line L260 (813.3607, -63.5) -> (813.3607, -50.8)
  arc A160 (813.3607, -63.5) -> (818.4407, -63.5) centre (815.9007, -63.5) ccw
  arc A161 (818.4407, -50.8) -> (813.3607, -50.8) centre (815.9007, -50.8) ccw
  line L261 (841.348, -58.42) -> (841.348, -57.15) construction
  line L262 (843.888, -63.5) -> (843.888, -50.8)
  line L263 (838.808, -63.5) -> (838.808, -50.8)
  arc A162 (838.808, -63.5) -> (843.888, -63.5) centre (841.348, -63.5) ccw
  arc A163 (843.888, -50.8) -> (838.808, -50.8) centre (841.348, -50.8) ccw
  line L264 (866.7953, -58.42) -> (866.7953, -57.15) construction
  line L265 (869.3353, -63.5) -> (869.3353, -50.8)
  line L266 (864.2553, -63.5) -> (864.2553, -50.8)
  arc A164 (864.2553, -63.5) -> (869.3353, -63.5) centre (866.7953, -63.5) ccw
  arc A165 (869.3353, -50.8) -> (864.2553, -50.8) centre (866.7953, -50.8) ccw
  line L267 (892.2426, -58.42) -> (892.2426, -57.15) construction
  line L268 (894.7826, -63.5) -> (894.7826, -50.8)
  line L269 (889.7026, -63.5) -> (889.7026, -50.8)
  arc A166 (889.7026, -63.5) -> (894.7826, -63.5) centre (892.2426, -63.5) ccw
  arc A167 (894.7826, -50.8) -> (889.7026, -50.8) centre (892.2426, -50.8) ccw
  line L270 (917.6898, -58.42) -> (917.6898, -57.15) construction
  line L271 (920.2298, -63.5) -> (920.2298, -50.8)
  line L272 (915.1498, -63.5) -> (915.1498, -50.8)
  arc A168 (915.1498, -63.5) -> (920.2298, -63.5) centre (917.6898, -63.5) ccw
  arc A169 (920.2298, -50.8) -> (915.1498, -50.8) centre (917.6898, -50.8) ccw
  line L273 (943.1371, -58.42) -> (943.1371, -57.15) construction
  line L274 (945.6771, -63.5) -> (945.6771, -50.8)
  line L275 (940.5971, -63.5) -> (940.5971, -50.8)
  arc A170 (940.5971, -63.5) -> (945.6771, -63.5) centre (943.1371, -63.5) ccw
  arc A171 (945.6771, -50.8) -> (940.5971, -50.8) centre (943.1371, -50.8) ccw
  line L276 (968.5844, -58.42) -> (968.5844, -57.15) construction
  line L277 (971.1244, -63.5) -> (971.1244, -50.8)
  line L278 (966.0444, -63.5) -> (966.0444, -50.8)
  arc A172 (966.0444, -63.5) -> (971.1244, -63.5) centre (968.5844, -63.5) ccw
  arc A173 (971.1244, -50.8) -> (966.0444, -50.8) centre (968.5844, -50.8) ccw
  line L279 (994.0317, -58.42) -> (994.0317, -57.15) construction
  line L280 (996.5717, -63.5) -> (996.5717, -50.8)
  line L281 (991.4917, -63.5) -> (991.4917, -50.8)
  arc A174 (991.4917, -63.5) -> (996.5717, -63.5) centre (994.0317, -63.5) ccw
  arc A175 (996.5717, -50.8) -> (991.4917, -50.8) centre (994.0317, -50.8) ccw
  line L282 (1019.479, -58.42) -> (1019.479, -57.15) construction
  line L283 (1022.019, -63.5) -> (1022.019, -50.8)
  line L284 (1016.939, -63.5) -> (1016.939, -50.8)
  arc A176 (1016.939, -63.5) -> (1022.019, -63.5) centre (1019.479, -63.5) ccw
  arc A177 (1022.019, -50.8) -> (1016.939, -50.8) centre (1019.479, -50.8) ccw
  line L285 (1044.9263, -58.42) -> (1044.9263, -57.15) construction
  line L286 (1047.4663, -63.5) -> (1047.4663, -50.8)
  line L287 (1042.3863, -63.5) -> (1042.3863, -50.8)
  arc A178 (1042.3863, -63.5) -> (1047.4663, -63.5) centre (1044.9263, -63.5) ccw
  arc A179 (1047.4663, -50.8) -> (1042.3863, -50.8) centre (1044.9263, -50.8) ccw
  line L288 (1070.3736, -58.42) -> (1070.3736, -57.15) construction
  line L289 (1072.9136, -63.5) -> (1072.9136, -50.8)
  line L290 (1067.8336, -63.5) -> (1067.8336, -50.8)
  arc A180 (1067.8336, -63.5) -> (1072.9136, -63.5) centre (1070.3736, -63.5) ccw
  arc A181 (1072.9136, -50.8) -> (1067.8336, -50.8) centre (1070.3736, -50.8) ccw
  line L291 (1095.8209, -58.42) -> (1095.8209, -57.15) construction
  line L292 (1098.3609, -63.5) -> (1098.3609, -50.8)
  line L293 (1093.2809, -63.5) -> (1093.2809, -50.8)
  arc A182 (1093.2809, -63.5) -> (1098.3609, -63.5) centre (1095.8209, -63.5) ccw
  arc A183 (1098.3609, -50.8) -> (1093.2809, -50.8) centre (1095.8209, -50.8) ccw
  line L294 (1121.2681, -58.42) -> (1121.2681, -57.15) construction
  line L295 (1123.8081, -63.5) -> (1123.8081, -50.8)
  line L296 (1118.7281, -63.5) -> (1118.7281, -50.8)
  arc A184 (1118.7281, -63.5) -> (1123.8081, -63.5) centre (1121.2681, -63.5) ccw
  arc A185 (1123.8081, -50.8) -> (1118.7281, -50.8) centre (1121.2681, -50.8) ccw
  line L297 (1146.7154, -58.42) -> (1146.7154, -57.15) construction
  line L298 (1149.2554, -63.5) -> (1149.2554, -50.8)
  line L299 (1144.1754, -63.5) -> (1144.1754, -50.8)
  arc A186 (1144.1754, -63.5) -> (1149.2554, -63.5) centre (1146.7154, -63.5) ccw
  arc A187 (1149.2554, -50.8) -> (1144.1754, -50.8) centre (1146.7154, -50.8) ccw
  line L300 (1172.1627, -58.42) -> (1172.1627, -57.15) construction
  line L301 (1174.7027, -63.5) -> (1174.7027, -50.8)
  line L302 (1169.6227, -63.5) -> (1169.6227, -50.8)
  arc A188 (1169.6227, -63.5) -> (1174.7027, -63.5) centre (1172.1627, -63.5) ccw
  arc A189 (1174.7027, -50.8) -> (1169.6227, -50.8) centre (1172.1627, -50.8) ccw
  line L303 (1197.61, -58.42) -> (1197.61, -57.15) construction
  line L304 (1200.15, -63.5) -> (1200.15, -50.8)
  line L305 (1195.07, -63.5) -> (1195.07, -50.8)
  arc A190 (1195.07, -63.5) -> (1200.15, -63.5) centre (1197.61, -63.5) ccw
  arc A191 (1200.15, -50.8) -> (1195.07, -50.8) centre (1197.61, -50.8) ccw
  point P0 (-1168.9877, -48.26)
  point P1 (-1143.5404, -48.26)
  point P2 (-1118.0931, -48.26)
  point P3 (-1092.6459, -48.26)
  point P4 (-1067.1986, -48.26)
  point P5 (-1041.7513, -48.26)
  point P6 (-1016.304, -48.26)
  point P7 (-990.8567, -48.26)
  point P8 (-965.4094, -48.26)
  point P9 (-939.9621, -48.26)
  point P10 (-914.5148, -48.26)
  point P11 (-889.0676, -48.26)
  point P12 (-863.6203, -48.26)
  point P13 (-838.173, -48.26)
  point P14 (-812.7257, -48.26)
  point P15 (-787.2784, -48.26)
  point P16 (-761.8311, -48.26)
  point P17 (-736.3838, -48.26)
  point P18 (-710.9365, -48.26)
  point P19 (-685.4893, -48.26)
  point P20 (-660.042, -48.26)
  point P21 (-634.5947, -48.26)
  point P22 (-609.1474, -48.26)
  point P23 (-583.7001, -48.26)
  point P24 (-558.2528, -48.26)
  point P25 (-532.8055, -48.26)
  point P26 (-507.3582, -48.26)
  point P27 (-481.911, -48.26)
  point P28 (-456.4637, -48.26)
  point P29 (-431.0164, -48.26)
  point P30 (-405.5691, -48.26)
  point P31 (-380.1218, -48.26)
  point P32 (-354.6745, -48.26)
  point P33 (-329.2272, -48.26)
  point P34 (-303.7799, -48.26)
  point P35 (-278.3327, -48.26)
  point P36 (-252.8854, -48.26)
  point P37 (-227.4381, -48.26)
  point P38 (-201.9908, -48.26)
  point P39 (-176.5435, -48.26)
  point P40 (-151.0962, -48.26)
  point P41 (-125.6489, -48.26)
  point P42 (-100.2016, -48.26)
  point P43 (-74.7544, -48.26)
  point P44 (-49.3071, -48.26)
  point P45 (-23.8598, -48.26)
  point P46 (1.5875, -48.26)
  point P47 (27.0348, -48.26)
  point P48 (52.4821, -48.26)
  point P49 (77.9294, -48.26)
  point P50 (103.3766, -48.26)
  point P51 (128.8239, -48.26)
  point P52 (154.2712, -48.26)
  point P53 (179.7185, -48.26)
  point P54 (205.1658, -48.26)
  point P55 (230.6131, -48.26)
  point P56 (256.0604, -48.26)
  point P57 (281.5077, -48.26)
  point P58 (306.9549, -48.26)
  point P59 (332.4022, -48.26)
  point P60 (357.8495, -48.26)
  point P61 (383.2968, -48.26)
  point P62 (408.7441, -48.26)
  point P63 (434.1914, -48.26)
  point P64 (459.6387, -48.26)
  point P65 (485.086, -48.26)
  point P66 (510.5332, -48.26)
  point P67 (535.9805, -48.26)
  point P68 (561.4278, -48.26)
  point P69 (586.8751, -48.26)
  point P70 (612.3224, -48.26)
  point P71 (637.7697, -48.26)
  point P72 (663.217, -48.26)
  point P73 (688.6643, -48.26)
  point P74 (714.1115, -48.26)
  point P75 (739.5588, -48.26)
  point P76 (765.0061, -48.26)
  point P77 (790.4534, -48.26)
  point P78 (815.9007, -48.26)
  point P79 (841.348, -48.26)
  point P80 (866.7953, -48.26)
  point P81 (892.2426, -48.26)
  point P82 (917.6898, -48.26)
  point P83 (943.1371, -48.26)
  point P84 (968.5844, -48.26)
  point P85 (994.0317, -48.26)
  point P86 (1019.479, -48.26)
  point P87 (1044.9263, -48.26)
  point P88 (1070.3736, -48.26)
  point P89 (1095.8209, -48.26)
  point P90 (1121.2681, -48.26)
  point P91 (1146.7154, -48.26)
  point P92 (1172.1627, -48.26)
  point P93 (1197.61, -48.26)
  dimension "d37" = 5.08
  dimension "d38" = 5.08
  dimension "d39" = 19.05
  dimension "d42" = 2392.045
  dimension "d43" = 0
  constraint coincident L1 L4.end
  constraint perpendicular L1 L4
  constraint coincident L11 L22.end
  constraint perpendicular L11 L22
  constraint tangent L19 A2
  constraint tangent L20 A2
  constraint coincident A2 L22.start
  constraint collinear L21 L22
  constraint midpoint L2 L23.start
  constraint perpendicular L2 L23
  measures "d37" diameter of A2
  measures "d38" diameter of A3
  measures "d39" distance of L23.start L23.end
split "Split1" by plane through (0, 0, 0) normal (1, 0, 0) bodies 1 makes body 4 at (402.8732, 3.175, -33.8667)
mirror "Mirror1" about plane through (0, 0, 0) normal (1, 0, 0) of bodies 4 merged
delete_body "RemoveBody1" bodies 1
split "Split2" by plane through (1216.025, 0, 0) normal (-1, 0, 0) bodies 4 makes body 5 at (402.8732, 3.175, -67.7333)
split "Split3" by plane through (-1216.025, 0, 0) normal (1, 0, 0) bodies 5 makes body 6 at (402.8732, 3.175, -67.7333)
split "Split4" by plane through (0, 3.175, 0) normal (0, -1, 0) bodies 6 makes body 7 at (-1213.7911, 0.51, -33.8807) makes body 8 at (1213.7911, 0.51, -33.8807)
shell "Shell1" thickness 3.175 removed faces 2 at (1216.025, 40.005, -83.82) at (-1216.025, 40.005, -83.82) on bodies 6
combine "Combine1" operation add target body 6 tool bodies 4 5 7 8
extrude "Extrude7" cut sketch "Sketch7" against normal blind 20.32 contours L19 L20 A2 A3 | L25 L26 A4 A5 | L28 L29 A6 A7 | L31 L32 A8 A9 | L34 L35 A10 A11 | L37 L38 A12 A13 | L40 L41 A14 A15 | L43 L44 A16 A17 | L46 L47 A18 A19 | L49 L50 A20 A21 | L52 L53 A22 A23 | L55 L56 A24 A25 | L58 L59 A26 A27 | L61 L62 A28 A29 | L64 L65 A30 A31 | L67 L68 A32 A33 | L70 L71 A34 A35 | L73 L74 A36 A37 | L76 L77 A38 A39 | L79 L80 A40 A41 | L82 L83 A42 A43 | L85 L86 A44 A45 | L88 L89 A46 A47 | L91 L92 A48 A49 | L94 L95 A50 A51 | L97 L98 A52 A53 | L100 L101 A54 A55 | L103 L104 A56 A57 | L106 L107 A58 A59 | L109 L110 A60 A61 | L112 L113 A62 A63 | L115 L116 A64 A65 | L118 L119 A66 A67 | L121 L122 A68 A69 | L124 L125 A70 A71 | L127 L128 A72 A73 | L130 L131 A74 A75 | L133 L134 A76 A77 | L136 L137 A78 A79 | L139 L140 A80 A81 | L142 L143 A82 A83 | L145 L146 A84 A85 | L148 L149 A86 A87 | L151 L152 A88 A89 | L154 L155 A90 A91 | L157 L158 A92 A93 | L160 L161 A94 A95 | L163 L164 A96 A97 | L166 L167 A98 A99 | L169 L170 A100 A101 | L172 L173 A102 A103 | L175 L176 A104 A105 | L178 L179 A106 A107 | L181 L182 A108 A109 | L184 L185 A110 A111 | L187 L188 A112 A113 | L190 L191 A114 A115 | L193 L194 A116 A117 | L196 L197 A118 A119 | L199 L200 A120 A121 | L202 L203 A122 A123 | L205 L206 A124 A125 | L208 L209 A126 A127 | L211 L212 A128 A129 | L214 L215 A130 A131 | L217 L218 A132 A133 | L220 L221 A134 A135 | L223 L224 A136 A137 | L226 L227 A138 A139 | L229 L230 A140 A141 | L232 L233 A142 A143 | L235 L236 A144 A145 | L238 L239 A146 A147 | L241 L242 A148 A149 | L244 L245 A150 A151 | L247 L248 A152 A153 | L250 L251 A154 A155 | L253 L254 A156 A157 | L256 L257 A158 A159 | L259 L260 A160 A161 | L262 L263 A162 A163 | L265 L266 A164 A165 | L268 L269 A166 A167 | L271 L272 A168 A169 | L274 L275 A170 A171 | L277 L278 A172 A173 | L280 L281 A174 A175 | L283 L284 A176 A177 | L286 L287 A178 A179 | L289 L290 A180 A181 | L292 L293 A182 A183 | L295 L296 A184 A185 | L298 L299 A186 A187 | L301 L302 A188 A189 | L304 L305 A190 A191 bodies 6